Autodesk Fusion 360 part; units mm, degrees
note: some values were not read from the file. Set by a fixed rule: which sketch regions a step uses.
(part 2 of 2)
sketch "Sketch13" plane through (0, 0, 3.5) normal (0, 0, 1) x (-1, 0, 0) in component "bumper_vertical"
  line L0 (10, -28.8) -> (-10, -28.8)
  line L1 (-10, -28.8) -> (-10, -34.4)
  line L2 (-10, -34.4) -> (10, -34.4)
  line L3 (10, -34.4) -> (10, -28.8)
  line L4 (10, -34.4) -> (-10, -34.4)
  line L5 (-10, -34.4) -> (-10, -32.9)
  line L6 (-10, -32.9) -> (10, -32.9)
  line L7 (10, -32.9) -> (10, -34.4)
  line L8 (10, -28.8) -> (-10.0749, -28.8)
  line L9 (-10.0749, -28.8) -> (-10.0749, -30.3)
  line L10 (-10.0749, -30.3) -> (10, -30.3)
  line L11 (10, -30.3) -> (10, -28.8)
  dimension "d268" = 1.5
  dimension "d271" = 1.5
  constraint horizontal L4
  constraint vertical L5
  constraint horizontal L6
  constraint vertical L7
  constraint coincident L1 L5.end
  constraint coincident L2.end L3.start
  constraint horizontal L8
  constraint vertical L9
  constraint horizontal L10
  constraint vertical L11
  constraint coincident L0.start L3.end
  measures "d268" distance of L0.start L10.end
  measures "d271" distance of L4 L6
sketch "Sketch14" plane through (0, 0, 3.5) normal (0, 0, 1) x (-1, 0, 0) in component "bumper_vertical"
  line L0 (10, 29) -> (10, 34.4)
  line L1 (10, 34.4) -> (-10, 34.4)
  line L2 (-10, 34.4) -> (-10, 29)
  line L3 (-10, 29) -> (10, 29)
  line L4 (10, 34.4) -> (-10.0697, 34.4)
  line L5 (-10.0697, 34.4) -> (-10.0697, 32.9)
  line L6 (-10.0697, 32.9) -> (10, 32.9)
  line L7 (10, 32.9) -> (10, 34.4)
  line L8 (10, 29) -> (-10.0708, 29)
  line L9 (-10.0708, 29) -> (-10.0708, 30.5)
  line L10 (-10.0708, 30.5) -> (10, 30.5)
  line L11 (10, 30.5) -> (10, 29)
  dimension "d269" = 1.5
  dimension "d270" = 1.5
  constraint horizontal L4
  constraint vertical L5
  constraint horizontal L6
  constraint vertical L7
  constraint coincident L0.end L1.start
  constraint horizontal L8
  constraint vertical L9
  constraint horizontal L10
  constraint vertical L11
  constraint coincident L0.start L3.end
  measures "d269" distance of L0.end L6.end
  measures "d270" distance of L0.start L10.end
extrude "Extrude6" [suppressed] in component "bumper_vertical"
component "bracket_omni_wheel" placed x (1, 0, 0) y (0, 1, 0) z (0, 0, 1) at (0, 0, 0)
component "chassis_bottom_deck" placed x (1, 0, 0) y (0, 1, 0) z (0, 0, 1) at (0, 0, 0)
component "chassis_top_deck" placed x (1, 0, 0) y (0, 1, 0) z (0, 0, 1) at (0, 0, 0)
component "deck_vertical_spacer" placed x (1, 0, 0) y (0, 1, 0) z (0, 0, 1) at (0, 0, 0)
component "component_spacer" placed x (1, 0, 0) y (0, 1, 0) z (0, 0, 1) at (0, 0, 0)
component "profile_square" placed x (1, 0, 0) y (0, 1, 0) z (0, 0, 1) at (0, 0, 0)
component "profile_rectangle" placed x (1, 0, 0) y (0, 1, 0) z (0, 0, 1) at (0, 0, 0)
component "profile_switch" placed x (1, 0, 0) y (0, 1, 0) z (0, 0, 1) at (0, 0, 0)
component "side_bracket_1" placed x (1, 0, 0) y (0, 1, 0) z (0, 0, 1) at (6.1728, 22.7991, -24.75) in component "bracket_omni_wheel"
component "side_bracket_2" placed x (-1, 0, 0) y (0, -1, 0) z (0, 0, 1) at (-30.6295, -31.9665, -27.6629) in component "bracket_omni_wheel"
component "top_bracket" placed x (1, 0, 0) y (0, 1, 0) z (0, 0, 1) at (0, 0, 0) in component "bracket_omni_wheel"
equation "thickness = 3 mm" comment "bracket thickness"
equation "wheel_radius = 24 mm"
equation "wheel_width = 25.9 mm"
equation "washer_width = 1 mm"
equation "M3_diameter = 3 mm"
equation "d6 = wheel_width + 2 * washer_width + tolerance + 2 * thickness"
equation "tolerance = 0.5 mm"
equation "d8 = bracket_width"
equation "bracket_width = 22 mm"
equation "d11 = d10"
equation "d12 = M3_diameter + tolerance"
equation "d13 = d12"
equation "d14 = d12"
equation "d15 = d12"
equation "d16 = bracket_width"
equation "d17 = bracket_side_hole_height - thickness + 8 mm"
equation "chassis_clearance = 68.5 mm"
equation "bracket_side_hole_height = chassis_clearance - wheel_radius"
equation "d20 = 7 mm + tolerance"
equation "d21 = bracket_side_hole_height - thickness"
equation "d22 = thickness"
equation "d24 = 8 mm + tolerance"
equation "d29 = thickness"
equation "d42 = chassis_lenght"
equation "d43 = chassis_width"
equation "d54 = wheel_width"
equation "d55 = wheel_radius * 2"
equation "d58 = d56"
equation "d59 = d57"
equation "d62 = M3_diameter"
equation "d63 = M3_diameter"
equation "d64 = M3_diameter"
equation "d65 = M3_diameter"
equation "d66 = M3_diameter"
equation "d67 = M3_diameter"
equation "d68 = M3_diameter"
equation "d69 = M3_diameter"
equation "d70 = d50"
equation "d71 = d51"
equation "d72 = d53"
equation "d73 = d52"
equation "chassis_width = 300 mm"
equation "chassis_lenght = 300 mm"
equation "d78 = chassis_lenght"
equation "d79 = chassis_width"
equation "d80 = ( 0.7 * 56 ) * 1 mm"
equation "d88 = vertical_support_ext_diameter"
equation "vertical_support_ext_diameter = 10 mm"
equation "vertical_support_hole = 4 mm + tolerance"
equation "d119 = d120"
equation "d121 = d122"
equation "d125 = d126"
equation "d137 = d136"
equation "d138 = d136"
equation "d142 = d141"
equation "d143 = d141"
equation "d168 = d169"
equation "d170 = 12 mm + 9 mm"
equation "d178 = d177"
equation "d179 = d177"
equation "d180 = d177"
equation "d181 = d177"
equation "d202 = M3_diameter + tolerance"
equation "d203 = M3_diameter + tolerance"
equation "d204 = M3_diameter + tolerance"
equation "d205 = M3_diameter + tolerance"
equation "d210 = d209"
equation "d225 = d224"
equation "d230 = d226"
equation "d251 = 60 mm + ( 1.5 * 2 ) * 1 mm + ( 2.9 * 2 ) * 1 mm"
equation "d263 = ( 1.5 * 2 ) * 1 mm + 2.4 mm"
equation "d265 = ( 1.5 * 2 ) * 1 mm + 2.6 mm"
equation "d279 = d278"
equation "d280 = d278"
equation "d296 = d295"
equation "d297 = d295"
equation "d298 = d295"
named bodies: "side_bracket_1", "side_bracket_2", "top_bracket", "chassis_bottom_deck", "top_mast"
